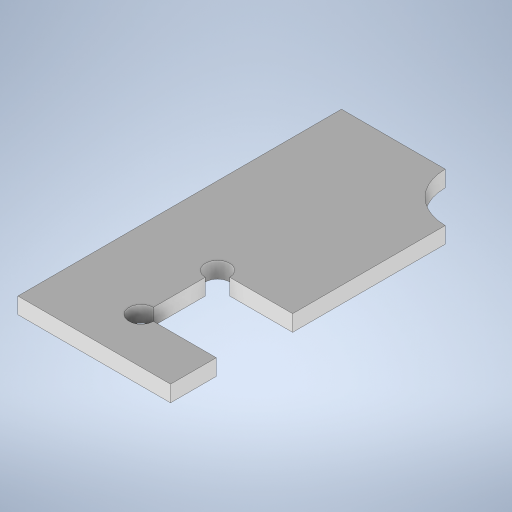
# Autodesk Inventor part: bendpart_90deg
Saved by Autodesk Inventor 2024 (Build 280153000, 153)
## iProperties
Created: 2025-02-17
Part Number: bendpart_90deg
Material: 一般
Document SubType Name: Modeling
Designer: tanoue_kota
Density: 1 g/cm^3
Appearance: 既定
Author: tanoue_kota
Autodesk Inventor part; units mm, degrees
ref_plane "YZ Plane" through (0, 0, 0) normal (1, 0, 0) x (0, 1, 0)
ref_plane "XZ Plane" through (0, 0, 0) normal (0, 1, 0) x (-1, 0, 0)
ref_plane "XY Plane" through (0, 0, 0) normal (0, 0, 1) x (1, 0, 0)
sketch "スケッチ1" plane through (0, 0, 0) normal (0, 1, 0) x (-1, 0, 0)
  line L0 (0, 0) -> (25, 0)
  line L1 (25, 0) -> (25, -33)
  line L2 (25, -33) -> (0, -33)
  line L3 (0, -33) -> (0, 0)
  line L4 (25, -27) -> (0, -33)
  dimension "d0" = 33
  dimension "d1" = 25
  dimension "d2" = 27
  constraints: 10 end point, 2 parallel, 1 horizontal, 1 perpendicular, 1 point on line
  measures "d0" distance of L2.end L0.start
  measures "d1" distance of L0.start L0.end
  measures "d2" distance from line of L0 L4.start
extrude "押し出し1" add sketch "スケッチ1" along normal blind 2.65
sketch "スケッチ2" plane through (0, 2.65, 0) normal (0, 1, 0) x (1, 0, 0)
  line L0 (0, 0) -> (0, 33) projected
  circle A0 centre (0, 33) radius 8
  dimension "d5" = 16
  constraints: 1 centre point
  measures "d5" diameter of A0
extrude "押し出し2" cut sketch "スケッチ2" against normal blind 2.65
sketch "スケッチ3" plane through (0, 2.65, 0) normal (0, 1, 0) x (1, 0, 0)
  line L0 (-25, 0) -> (0, 0) projected
  line L1 (-25, 0) -> (-12.3, 0)
  line L2 (-12.3, 0) -> (-12.3, -20)
  line L3 (-12.3, -20) -> (-25, -20)
  line L4 (-25, -20) -> (-25, 0)
  line L5 (0, 0) -> (0, 25) projected
  circle A0 centre (-12.3, 0) radius 2
  point P0 (-12.3, -2)
  point P1 (-14.3, 0)
  dimension "d8" = 20
  dimension "d9" = 12.3
  dimension "d10" = 4
  constraints: 8 end point, 2 parallel, 1 centre point, 1 coincident, 1 horizontal, 1 perpendicular
  measures "d8" distance of L1.end L2.end
  measures "d9" distance between parallel lines of L5 L2
  measures "d10" diameter of A0
extrude "押し出し3" add sketch "スケッチ3" against normal blind 2.65 contours A0 L2 L3 L4 L0
sketch "スケッチ4" plane through (0, 2.65, 0) normal (0, 1, 0) x (1, 0, 0)
  arc A0 (-14.3, 0) -> (-12.3, -2) centre (-12.3, 0) ccw projected
  line L0 (-12.3, -2) -> (-12.3, -20) projected
  circle A1 centre (-12.3, 0) radius 2
  point P0 (0, 0)
  point P1 (-14.3, 0)
  constraints: 1 coincident, 3 other
extrude "押し出し4" cut sketch "スケッチ4" against normal blind 2.65
sketch "スケッチ5" plane through (0, 2.65, 0) normal (0, 1, 0) x (1, 0, 0)
  line L0 (-25, -20) -> (-12.3, -20) projected
  line L1 (-12.3, -20) -> (0, -20)
  line L2 (0, -20) -> (0, -12.5)
  line L3 (0, -12.5) -> (-12.3, -12.5)
  line L4 (-12.3, -12.5) -> (-12.3, -20)
  line L5 (-10.3, 0) -> (0, 0) projected
  dimension "d15" = 12.5
  dimension "d16" = 12.3
  constraints: 8 end point, 2 parallel, 1 horizontal, 1 perpendicular
  measures "d15" distance between parallel lines of L5 L3
  measures "d16" distance of L0.end L1.end
extrude "押し出し5" add sketch "スケッチ5" against normal blind 2.65
sketch "スケッチ6" plane through (0, 2.65, 0) normal (0, 1, 0) x (1, 0, 0)
  line L0 (-12.3, -12.5) -> (-12.3, -2) projected
  point P0 (0, 0)
hole "穴1" at (-12.3, 2.65, 12.5) direction (0, -1, 0) diameter 4 end through all
